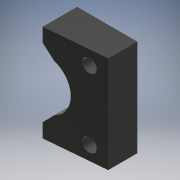
# Autodesk Inventor part: hotend_holder_clamp
Saved by Autodesk Inventor 2018 (Build 220112000, 112)
## iProperties
Created: 2018-07-15
Part Number: hotend_holder_clamp
Material: ABS Plastic
Document SubType Name: Modeling
Designer: Z. Deniz
Density: 1.06 g/cm^3
Appearance: Smooth - White
Author: Z. Deniz
Autodesk Inventor part; units mm, degrees
ref_plane "YZ Plane" through (0, 0, 0) normal (1, 0, 0) x (0, 1, 0)
ref_plane "XZ Plane" through (0, 0, 0) normal (0, 1, 0) x (-1, 0, 0)
ref_plane "XY Plane" through (0, 0, 0) normal (0, 0, 1) x (1, 0, 0)
sketch "Sketch1" plane through (0, 0, 0) normal (0, 1, 0) x (-1, 0, 0)
  arc A0 (6, -2.425) -> (6, -5.575) centre (6, -4) ccw construction
  line L0 (6, -2.425) -> (8, -2.425) construction
  arc A1 (8, -5.575) -> (8, -2.425) centre (8, -4) ccw construction
  line L1 (8, -5.575) -> (6, -5.575) construction
  arc A2 (6, -18.425) -> (6, -21.575) centre (6, -20) ccw construction
  line L2 (6, -18.425) -> (8, -18.425) construction
  arc A3 (8, -21.575) -> (8, -18.425) centre (8, -20) ccw construction
  line L3 (8, -21.575) -> (6, -21.575) construction
  line L4 (18, 0) -> (18, -4)
  line L5 (2, 0) -> (18, 0)
  line L6 (2, -24) -> (2, 0)
  line L7 (18, -24) -> (2, -24)
  line L8 (18, -20) -> (18, -24)
  arc A4 (18, -6) -> (18, -18) centre (18, -12) ccw
  line L9 (18, -6) -> (18, -4)
  line L10 (18, -20) -> (18, -18)
  arc A5 (18, -4) -> (18, -20) centre (18, -12) ccw
  circle A6 centre (8, -20) radius 2.375
  circle A7 centre (8, -4) radius 2.375
  point P0 (0, 0)
  point P1 (0, 0)
  dimension "d0" = 16
  dimension "d2" = 8
  dimension "d4" = 6
  dimension "d5" = 1.575
  dimension "d6" = 2
  dimension "d7" = 1.575
  dimension "d8" = 2
  dimension "d11" = 4.75
  dimension "d12" = 4.75
  constraints: 22 end point, 12 point on circle, 8 centre point, 2 coincident, 1 point on line, 1 other
  measures "d0" distance of L7.start L6.start
  measures "d2" radius of A5
  measures "d4" radius of A4
  measures "d5" radius of A3
  measures "d6" distance of A2.centre A3.centre
  measures "d7" radius of A1
  measures "d8" distance of A0.centre A1.centre
  measures "d11" diameter of A6
  measures "d12" diameter of A7
extrude "Extrusion1" add sketch "Sketch1" along normal blind 8 contours L4 A5 L8 L7 L6 L5
extrude "Extrusion2" add sketch "Sketch1" along normal blind 6 contours L9 A4 L10 A5
extrude "Extrusion3" add sketch "Sketch1" along normal blind 3 contours A6 | A7
sketch "Sketch2" plane through (-8, 3, -4) normal (0, 1, 0) x (1, 0, 0)
  circle A0 centre (0, 0) radius 2.375 projected
  circle A1 centre (0, 16) radius 2.375 projected
  circle A2 centre (0, 0) radius 2.375 projected
  circle A3 centre (0, 0) radius 1.575
  circle A4 centre (0, 16) radius 1.575
  point P0 (8, -4)
  dimension "d19" = 3.15
  dimension "d20" = 3.15
  constraints: 2 centre point, 2 coincident
  measures "d19" diameter of A3
  measures "d20" diameter of A4
extrude "Extrusion4" cut sketch "Sketch2" against normal through all contours A3 | A4
sketch "Sketch3" plane through (-18, 0, 0) normal (0, 0, 1) x (1, 0, 0)
  line L0 (0, 0) -> (16, 0) projected
  line L1 (16, 0) -> (16, 8) projected
  line L2 (0, 8) -> (16, 8) projected
  line L3 (0, 0) -> (0, 8) projected
  line L4 (8.425, 3) -> (8.425, 0) projected
  line L5 (16, 0) -> (0, 0) projected
  line L6 (0, 0) -> (0, 8) projected
  line L7 (16, 8) -> (0, 8) projected
  line L8 (16, 0) -> (16, 8) projected
  point P0 (18, 0)
sketch "Sketch4" plane through (-2, 0, -24) normal (0, 0, -1) x (-1, 0, 0)
  line L0 (0, 0) -> (16, 0) projected
  line L1 (16, 0) -> (16, 8) projected
  line L2 (0, 8) -> (16, 8) projected
  line L3 (0, 0) -> (0, 8) projected
  point P0 (-2, 0)
extrude "Extrusion6" cut sketch "Sketch3" against normal blind 0.25
extrude "Extrusion7" cut sketch "Sketch4" against normal blind 0.25
sketch "Sketch5" plane through (-2, 0, -0.25) normal (1, 0, 0) x (0, 0, -1)
  line L0 (23.5, 0) -> (23.5, 8) projected
  line L1 (0, 8) -> (23.5, 8) projected
  line L2 (0, 8) -> (0, 0) projected
  line L3 (0, 0) -> (23.5, 0) projected
  point P0 (-0.25, 0)
extrude "Extrusion8" cut sketch "Sketch5" against normal blind 2
chamfer "Chamfer1" distance 2 distance2 2.5 1 edges at (-18, 3, -18) measured on face at (-18, 3, -18.5)
chamfer "Chamfer2" distance 2.5 distance2 2 1 edges at (-18, 3, -6) measured on face at (-17.5017, 3, -6.0207)
sketch "Sketch11" plane through (-2, 0, -23.75) normal (0, 0, -1) x (-1, 0, 0)
  line L0 (2, 8) -> (2, 0) projected
  line L1 (16, 0) -> (2, 0) projected
  line L2 (16, 8) -> (16, 0) projected
  line L3 (2, 8) -> (16, 8) projected
  line L4 (2, 0) -> (16, 0) projected
  line L5 (16, 0) -> (2, 1.2248)
  line L6 (2, 0) -> (2, 8) projected
  line L7 (16, 0) -> (30.0535, 0) construction
  point P0 (-2, 0)
  dimension "d46" = 175
  constraints: 4 end point, 1 equal length, 1 horizontal, 1 point on line
  measures "d46" angle of L7 L5
extrude "Extrusion11" cut sketch "Sketch11" against normal through all contours L5 L1 L0
sketch "Sketch12" plane through (-2, 0, -23.75) normal (0, 0, -1) x (-1, 0, 0)
  line L0 (2, 1.2248) -> (16, 0) projected
  line L1 (16, 8) -> (16, 0) projected
  line L2 (2, 8) -> (16, 8) projected
  line L3 (2, 8) -> (2, 1.2248) projected
  line L4 (16, 0) -> (2, 1.2248) projected
  line L5 (2, 1.2248) -> (2, 8) projected
  line L6 (16, 8) -> (2, 8) projected
  line L7 (16, 0) -> (16, 8) projected
  point P0 (-2, 0)
extrude "Extrusion12" cut sketch "Sketch12" against normal blind 0.5
sketch "Sketch13" plane through (-18, 0, -0.25) normal (0, 0, 1) x (1, 0, 0)
  line L0 (0, 0) -> (14, 1.2248) projected
  line L1 (14, 1.2248) -> (14, 8) projected
  line L2 (0, 8) -> (14, 8) projected
  line L3 (0, 0) -> (0, 8) projected
  point P0 (18, 0)
extrude "Extrusion13" cut sketch "Sketch13" against normal blind 0.5
equation "\"d12\" = d11"
body "Solid1"
